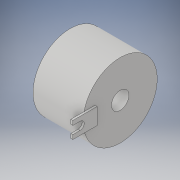
# Autodesk Inventor part: SlipRing
Saved by Autodesk Inventor 2019 (Build 230136000, 136)
## iProperties
Created: 2019-01-14
Part Number: SlipRing
Material: Generic
Document SubType Name: Modeling
Designer: nxgam
Density: 1 g/cm^3
Appearance: Default
Author: nxgam
Autodesk Inventor part; units mm, degrees
ref_plane "YZ Plane" through (0, 0, 0) normal (1, 0, 0) x (0, 1, 0)
ref_plane "XZ Plane" through (0, 0, 0) normal (0, 1, 0) x (-1, 0, 0)
ref_plane "XY Plane" through (0, 0, 0) normal (0, 0, 1) x (1, 0, 0)
sketch "Sketch1" plane through (0, 0, 0) normal (1, 0, 0) x (0, 1, 0)
  circle A0 centre (0, 0) radius 27.051
  dimension "d0" = 54.102
  constraints: 1 centre point, 1 coincident
  measures "d0" diameter of A0
extrude "Extrusion1" add sketch "Sketch1" along normal blind 36.576
sketch "Sketch2" plane through (36.576, 0, 0) normal (1, 0, 0) x (0, 0, -1)
  circle A0 centre (0, 0) radius 6.35
  dimension "d3" = 12.7
  constraints: 1 centre point, 1 coincident
  measures "d3" diameter of A0
extrude "Extrusion2" cut sketch "Sketch2" against normal through all
sketch "Sketch3" plane through (36.576, 0, 0) normal (1, 0, 0) x (0, 0, -1)
  circle A0 centre (0, 0) radius 6.35 projected
  circle A1 centre (0, 0) radius 27.051 projected
  line L0 (0, 0) -> (-36.068, 0) construction
  line L1 (-18.288, -6.0325) -> (-36.068, -6.0325)
  line L2 (-36.068, -6.0325) -> (-36.068, 6.0325)
  line L3 (-36.068, 6.0325) -> (-18.288, 6.0325)
  line L4 (-18.288, 6.0325) -> (-18.288, -6.0325)
  line L5 (-18.288, -6.0325) -> (-36.068, 6.0325) construction
  line L6 (-36.068, -6.0325) -> (-18.288, 6.0325) construction
  circle A2 centre (-30.734, 0) radius 2.921
  line L7 (-30.734, 2.921) -> (-36.068, 2.921)
  line L8 (-30.734, -2.921) -> (-36.068, -2.921)
  point P0 (-27.178, 0)
  dimension "d6" = 27.178
  dimension "d7" = 12.065
  dimension "d8" = 17.78
  dimension "d9" = 5.842
  dimension "d10" = 5.334
  constraints: 18 end point, 4 point on line, 3 midpoint, 3 parallel, 2 horizontal, 2 perpendicular, 2 point on circle, 2 tangent, 1 centre point
  measures "d6" distance of point (-27.178, 0) L0.start
  measures "d7" distance of L3.end L1.start
  measures "d8" distance of L2.end L3.end
  measures "d9" diameter of A2
  measures "d10" distance from line of L2 A2.centre
extrude "Extrusion3" add sketch "Sketch3" along normal blind 1.524 contours L3 L4 L1 A1 | A1 L1 L2 L8 A2 L7 L3 picked at (-21.1837, 0.6753)
body "Solid1"
